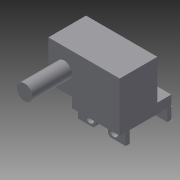
# Autodesk Inventor part: RearBearingMount
Saved by Autodesk Inventor 2015 (Build 190159000, 159)
## iProperties
Created: 2016-03-31
Part Number: RearBearingMount
Material: Generic
Document SubType Name: Modeling
Designer: Hatch
Density: 1 g/cm^3
Appearance: Default
Author: Hatch
Autodesk Inventor part; units mm, degrees
ref_plane "YZ Plane" through (0, 0, 0) normal (1, 0, 0) x (0, 1, 0)
ref_plane "XZ Plane" through (0, 0, 0) normal (0, 1, 0) x (-1, 0, 0)
ref_plane "XY Plane" through (0, 0, 0) normal (0, 0, 1) x (1, 0, 0)
sketch "Sketch1" plane through (0, 0, 0) normal (0, 1, 0) x (-1, 0, 0)
  line L0 (0, 0) -> (24, 0)
  line L1 (24, 0) -> (24, -24)
  line L2 (24, -24) -> (0, -24)
  line L3 (0, -24) -> (0, 0)
  dimension "d0" = 24
  dimension "d1" = 24
  constraints: 8 end point, 2 parallel, 1 horizontal, 1 perpendicular
  measures "d0" distance of L1.end L2.end
  measures "d1" distance of L0.end L1.end
extrude "Extrusion1" add sketch "Sketch1" along normal blind 5
sketch "Sketch2" plane through (0, 0, 0) normal (0, -1, 0) x (1, 0, 0)
  line L0 (0, 0) -> (0, -3)
  line L1 (0, 0) -> (0, -24) projected
  line L2 (-24, -24) -> (-24, 0) projected
  line L3 (0, -3) -> (-24, -3)
  line L4 (-24, -3) -> (-24, -5)
  line L5 (-24, -5) -> (0, -5)
  line L6 (0, -5) -> (0, -3)
  dimension "d4" = 3
  dimension "d5" = 2
  constraints: 10 end point, 2 parallel, 2 point on line, 1 horizontal, 1 perpendicular
  measures "d4" distance of L0.start L0.end
  measures "d5" distance of L4.end L3.end
extrude "Extrusion2" add sketch "Sketch2" along normal blind 6
sketch "Sketch3" plane through (-24, 0, -3) normal (0, 0, 1) x (1, 0, 0)
  line L0 (24, -6) -> (0, -6)
  line L1 (0, -6) -> (24, -6) projected
  line L2 (12, -6) -> (12, -5)
  line L3 (12, -5) -> (12, -2.875)
  circle A0 centre (12, -2.875) radius 2.125
  point P0 (24, 0)
  dimension "d8" = 1
  dimension "d11" = 2.125
  dimension "d12" = 4.25
  constraints: 6 end point, 2 vertical, 1 centre point, 1 coincident, 1 horizontal, 1 midpoint
  measures "d8" distance of L2.start L2.end
  measures "d11" distance of L2.end L3.end
  measures "d12" diameter of A0
sketch "Sketch4" plane through (0, 5, 0) normal (0, 1, 0) x (1, 0, 0)
  line L0 (-24, 24) -> (0, 24)
  line L1 (0, 24) -> (0, 26)
  line L2 (0, 26) -> (-24, 26)
  line L3 (-24, 26) -> (-24, 24)
  point P0 (0, 0)
  dimension "d13" = 2
  constraints: 8 end point, 2 parallel, 1 horizontal, 1 perpendicular
  measures "d13" distance of L1.end L0.end
extrude "Extrusion3" add sketch "Sketch4" against normal blind 11
sketch "Sketch5" plane through (0, 5, 0) normal (0, 1, 0) x (1, 0, 0)
  line L0 (-24, 5) -> (-24, 24) projected
  line L1 (0, 3) -> (-24, 3)
  line L2 (-24, 3) -> (-24, 9)
  line L3 (-24, 9) -> (0, 9)
  line L4 (0, 9) -> (0, 3)
  point P0 (0, 0)
  dimension "d16" = 6
  constraints: 8 end point, 2 parallel, 1 horizontal, 1 perpendicular, 1 point on line
  measures "d16" distance of L1.end L2.end
extrude "Extrusion4" add sketch "Sketch5" along normal blind 10
extrude "Extrusion6" cut sketch "Sketch3" against normal through all
pattern_linear "Rectangular Pattern1" count 3 spacing 6 along (-1, 0, 0) of "Extrusion6" first direction both ways yes
sketch "Sketch7" plane through (0, 5, -26) normal (0, 0, -1) x (-1, 0, 0)
  circle A0 centre (18, -7.875) radius 2.125 projected
  line L0 (15.875, -7.875) -> (14.125, -7.875)
  circle A1 centre (12, -7.875) radius 2.125 projected
  circle A2 centre (6, -7.875) radius 2.125 projected
  line L1 (8.125, -7.875) -> (9.875, -7.875)
  line L2 (15, -7.875) -> (15, -11)
  line L3 (24, -11) -> (0, -11) projected
  line L4 (9, -7.875) -> (9, -5)
  line L5 (0, -5) -> (24, -5) projected
  line L6 (15, -11) -> (9, -11)
  line L7 (9, -11) -> (9, -5)
  line L8 (9, -5) -> (15, -5)
  line L9 (15, -5) -> (15, -11)
  constraints: 16 end point, 4 point on line, 3 parallel, 2 horizontal, 2 horizontal alignment, 2 midpoint, 2 point on circle, 1 perpendicular, 1 vertical, 2 other
sketch "Sketch8" plane through (-24, 0, -3) normal (0, 0, 1) x (1, 0, 0)
  circle A0 centre (18, -2.875) radius 2.125 projected
  line L0 (15.875, -2.875) -> (14.125, -2.875)
  circle A1 centre (12, -2.875) radius 2.125 projected
  line L1 (9.875, -2.875) -> (8.125, -2.875)
  circle A2 centre (6, -2.875) radius 2.125 projected
  line L2 (0, -6) -> (24, -6) projected
  line L3 (9, -6) -> (9, 0)
  line L4 (24, 0) -> (0, 0) projected
  line L5 (15, -6) -> (15, 0)
  line L6 (15, -6) -> (9, -6)
  line L7 (9, -6) -> (9, 0)
  line L8 (9, 0) -> (15, 0)
  line L9 (15, 0) -> (15, -6)
  constraints: 16 end point, 6 point on line, 3 parallel, 2 horizontal, 2 horizontal alignment, 2 perpendicular, 2 point on circle, 2 other
extrude "Extrusion7" cut sketch "Sketch8" against normal blind 2 contours L5 L2 L3 L1 A1 L0 | L0 A1 L1 L3 L4 L5
sketch "Sketch9" plane through (0, -6, -3) normal (0, 0, 1) x (1, 0, 0)
  line L0 (-9, 6) -> (-9, 0) projected
  line L1 (-9, 0) -> (0, 0) projected
  circle A0 centre (-6, 3.125) radius 2.125 projected
  line L2 (-15, 0) -> (-15, 6) projected
  line L3 (-24, 0) -> (0, 0) projected
  circle A1 centre (-18, 3.125) radius 2.125 projected
  line L4 (-9, 0) -> (-7.5, 0)
  line L5 (-15, 0) -> (-16.5, 0)
  line L6 (-9, 0) -> (-9, 1.3884)
  arc A2 (-9, 1.3884) -> (-7.5, 0) centre (-6, 3.125) ccw
  line L7 (-15, 0) -> (-15, 1.3884)
  arc A3 (-16.5, 0) -> (-15, 1.3884) centre (-18, 3.125) ccw
  point P0 (0, 6)
  dimension "d33" = 1.5
  dimension "d34" = 1.5
  constraints: 8 end point, 4 point on circle, 4 point on line, 2 centre point, 2 coincident
  measures "d33" distance of L0.end L4.end
  measures "d34" distance of L2.start L5.end
extrude "Extrusion8" cut sketch "Sketch9" against normal blind 2 contours A2 L1 L0 | L3 A3 L2
sketch "Sketch10" plane through (0, 0, 0) normal (1, 0, 0) x (0, 0, -1)
  line L0 (9, 5) -> (19, 5)
  line L1 (19, 5) -> (19, 15)
  line L2 (19, 15) -> (9, 15)
  line L3 (9, 15) -> (9, 5)
  point P0 (0, 0)
  dimension "d37" = 10
  constraints: 8 end point, 2 parallel, 1 horizontal, 1 perpendicular
  measures "d37" distance of L2.end L1.end
extrude "Extrusion9" add sketch "Sketch10" against normal blind 24
sketch "Sketch11" plane through (0, 15, 0) normal (0, 1, 0) x (1, 0, 0)
  line L0 (0, 5) -> (0, 19)
  line L1 (0, 19) -> (-24, 19)
  line L2 (-24, 19) -> (-24, 3)
  line L3 (-24, 3) -> (0, 3)
  line L4 (0, 3) -> (0, 19)
  point P0 (0, 0)
  point P1 (-24, 5)
  constraints: 10 end point, 2 parallel, 1 horizontal, 1 perpendicular
extrude "Extrusion10" add sketch "Sketch11" along normal blind 10
sketch "Sketch13" plane through (0, 0, 0) normal (1, 0, 0) x (0, 0, -1)
  line L0 (3, 25) -> (19, 25)
  line L1 (19, 25) -> (19, 5)
  line L2 (19, 5) -> (3, 5)
  line L3 (3, 5) -> (3, 25)
  point P0 (0, 0)
  constraints: 8 end point, 2 parallel, 1 horizontal, 1 perpendicular
extrude "Extrusion11" add sketch "Sketch13" along normal blind 12
sketch "Sketch14" plane through (-24, 5, -3) normal (0, 0, 1) x (1, 0, 0)
  line L0 (24, 0) -> (24, 20)
  line L1 (0, 20) -> (36, 20) projected
  line L2 (24, 10) -> (32, 10)
  circle A0 centre (28, 10) radius 3.75
  point P0 (24, -5)
  dimension "d44" = 8
  dimension "d45" = 7.5
  constraints: 4 end point, 2 midpoint, 1 centre point, 1 horizontal, 1 point on line, 1 vertical
  measures "d44" distance of L2.start L2.end
  measures "d45" diameter of A0
extrude "Extrusion12" add sketch "Sketch14" along normal blind 20
sketch "Sketch15" plane through (-24, 0, 0) normal (-1, 0, 0) x (0, 0, 1)
  line L0 (-3, 25) -> (0, 25)
  line L1 (0, 25) -> (0, 5)
  line L2 (0, 5) -> (-3, 5)
  line L3 (-3, 5) -> (-3, 25)
  point P0 (0, 0)
  constraints: 8 end point, 2 parallel, 1 horizontal, 1 perpendicular
extrude "Extrusion13" add sketch "Sketch15" against normal blind 36
sketch "Sketch16" plane through (-24, 0, -3) normal (-1, 0, 0) x (0, 0, 1)
  line L0 (3, 25) -> (-16, 25)
  line L1 (-16, 25) -> (-16, 5)
  line L2 (-16, 5) -> (3, 5)
  line L3 (3, 5) -> (3, 25)
  point P0 (3, 0)
  constraints: 8 end point, 2 parallel, 1 horizontal, 1 perpendicular
extrude "Extrusion14" add sketch "Sketch16" along normal blind 12
sketch "Sketch17" plane through (-24, 0, 0) normal (0, 0, 1) x (1, 0, 0)
  line L0 (-12, 25) -> (-12, 5) projected
  line L1 (-12, 15) -> (-4, 15)
  circle A0 centre (-4, 15) radius 3.9
  point P0 (24, 0)
  dimension "d52" = 8
  dimension "d53" = 7.8
  constraints: 2 end point, 1 centre point, 1 coincident, 1 horizontal, 1 midpoint
  measures "d52" distance of L1.start L1.end
  measures "d53" diameter of A0
extrude "Extrusion15" add sketch "Sketch17" along normal blind 20
sketch "Sketch18" plane through (-24, 0, 0) normal (0, 0, 1) x (1, 0, 0)
  line L0 (24, 5) -> (36, 5)
  line L1 (36, 5) -> (36, 25)
  line L2 (36, 25) -> (24, 25)
  line L3 (24, 25) -> (24, 5)
  point P0 (24, 0)
  constraints: 8 end point, 2 parallel, 1 horizontal, 1 perpendicular
extrude "Extrusion16" cut sketch "Sketch18" along normal through all both and the other way through all
body "Solid1"
